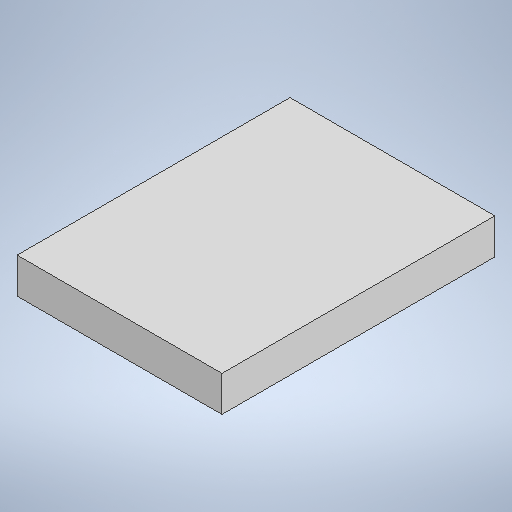
# Autodesk Inventor part: 2025_01_29_Reaktorkorpus_vorne
Saved by Autodesk Inventor 2025.1 (Build 291241000, 241)
## iProperties
Created: 2024-08-20
Part Number: 2025_01_29_Reaktorkorpus_vorne
Material: Generisch
Document SubType Name: Modeling
Designer: to86hug
Density: 1 g/cm^3
Appearance: Vorgabe
Author: to86hug
Autodesk Inventor part; units mm, degrees
ref_plane "YZ Plane" through (0, 0, 0) normal (1, 0, 0) x (0, 1, 0)
ref_plane "XZ Plane" through (0, 0, 0) normal (0, 1, 0) x (-1, 0, 0)
ref_plane "XY Plane" through (0, 0, 0) normal (0, 0, 1) x (1, 0, 0)
sketch "Skizze1" plane through (0, 0, 0) normal (0, 0, 1) x (1, 0, 0)
  line L0 (-67.75, 90.25) -> (67.75, 90.25)
  line L1 (67.75, 90.25) -> (67.75, -90.25)
  line L2 (67.75, -90.25) -> (-67.75, -90.25)
  line L3 (-67.75, -90.25) -> (-67.75, 90.25)
  line L4 (-67.75, 90.25) -> (67.75, -90.25) construction
  line L5 (67.75, 90.25) -> (-67.75, -90.25) construction
  point P0 (0, 0)
  dimension "d0" = 135.5
  dimension "d1" = 180.5
  constraints: 12 end point, 2 midpoint, 2 parallel, 1 horizontal, 1 perpendicular
  measures "d0" distance of L1.end L2.end
  measures "d1" distance of L0.end L1.end
extrude "Extrusion1" add sketch "Skizze1" along normal blind 23.5
